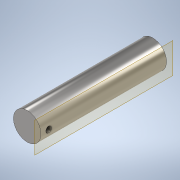
# Autodesk Inventor part: Part12
Saved by Autodesk Inventor 2020 (Build 240168000, 168)
## iProperties
Created: 2021-10-14
Part Number: Part12
Material: Steel, Mild
Document SubType Name: Modeling
Designer: simon.erikssonwestl
Density: 7.85 g/cm^3
Appearance: Semi-Polished
Author: simon.erikssonwestl
Autodesk Inventor part; units mm, degrees
ref_plane "XZ Plane" through (0, 0, 0) normal (0, 1, 0) x (-1, 0, 0)
ref_plane "XY Plane" through (0, 0, 0) normal (0, 0, 1) x (1, 0, 0)
sketch "Sketch1" plane through (0, 0, 0) normal (0, 0, 1) x (1, 0, 0)
  circle A0 centre (0, 0) radius 3.5
  dimension "d0" = 7
  constraints: 1 centre point, 1 coincident
  measures "d0" diameter of A0
extrude "Extrusion1" add sketch "Sketch1" along normal blind 32
ref_plane "Work Plane1" through (3.5, 0, 0) normal (1, 0, 0) x (0, 1, 0)
sketch "Sketch2" plane through (3.5, 0, 0) normal (1, 0, 0) x (0, 1, 0)
  line L0 (3.5, 32) -> (-3.5, 32) projected
  point P0 (0, 0)
  point P1 (0, 30)
  dimension "d3" = 2
  measures "d3" distance from line of point (0, 30) L0
hole "Hole1" at (3.5, 0, 30) direction (-1, 0, 0) diameter 1.5 depth 3.5 tip angle 118
body "Solid1"
